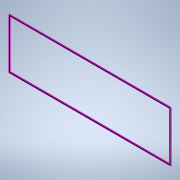
# Autodesk Inventor part: AluminumCasing
Saved by Autodesk Inventor 2021 (Build 250183000, 183)
## iProperties
Created: 2022-02-04
Part Number: AluminumCasing
Material: Generic
Document SubType Name: Modeling
Designer: tlar613
Density: 1 g/cm^3
Appearance: Default
Author: tlar613
Autodesk Inventor part; units mm, degrees
ref_plane "YZ Plane" through (0, 0, 0) normal (1, 0, 0) x (0, 1, 0)
ref_plane "XZ Plane" through (0, 0, 0) normal (0, 1, 0) x (-1, 0, 0)
ref_plane "XY Plane" through (0, 0, 0) normal (0, 0, 1) x (1, 0, 0)
sketch "Sketch1" plane through (0, 0, 0) normal (0, 0, 1) x (1, 0, 0)
  line L0 (-500, 150) -> (500, 150)
  line L1 (500, 150) -> (500, -150)
  line L2 (500, -150) -> (-500, -150)
  line L3 (-500, -150) -> (-500, 150)
  line L4 (-510, 160) -> (510, 160)
  line L5 (510, 160) -> (510, -160)
  line L6 (510, -160) -> (-510, -160)
  line L7 (-510, -160) -> (-510, 160)
  line L8 (0, 224) -> (0, -224) projected
  line L9 (-714, 0) -> (714, 0) projected
  point P0 (0, 0)
  dimension "d0" = 1000
  dimension "d1" = 300
  dimension "d2" = 1020
  dimension "d3" = 320
  constraints: 16 end point, 4 parallel, 2 horizontal, 2 perpendicular, 4 other
  measures "d0" distance of L0.start L0.end
  measures "d1" distance of L0.end L1.end
  measures "d2" distance of L4.start L4.end
  measures "d3" distance of L4.end L5.end
extrude "Extrusion1" add sketch "Sketch1" along normal blind 5 contours L3 L9 L7 L4 L8 L0 | L8 L4 L5 L9 L1 L0 | L3 L2 L8 L6 L7 L9 | L9 L5 L6 L8 L2 L1
body "Solid1"
